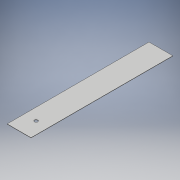
# Autodesk Inventor part: case
Saved by Autodesk Inventor 2019 (Build 230136000, 136)
## iProperties
Created: 2020-03-06
Part Number: case
Material: Generic
Document SubType Name: Sheet Metal
Designer: unusualgamer
Density: 1 g/cm^3
Sheet Metal Rule: Default_mm
Appearance: Default
Author: unusualgamer
Autodesk Inventor part; units mm, degrees
ref_plane "YZ Plane" through (0, 0, 0) normal (1, 0, 0) x (0, 1, 0)
ref_plane "XZ Plane" through (0, 0, 0) normal (0, 1, 0) x (-1, 0, 0)
ref_plane "XY Plane" through (0, 0, 0) normal (0, 0, 1) x (1, 0, 0)
sketch "Sketch1" plane through (0, 0, 0) normal (0, 1, 0) x (-1, 0, 0)
  line L0 (102.7304, -71.3481) -> (60.7304, -71.3481)
  line L1 (60.7304, -71.3481) -> (60.7304, 178.6519)
  line L2 (60.7304, 178.6519) -> (102.7304, 178.6519)
  line L3 (102.7304, 178.6519) -> (102.7304, -71.3481)
  point P0 (0, 0)
  dimension "d0" = 42
  dimension "d1" = 250
  measures "d0" distance of L1.end L2.end
  measures "d1" distance of L0.end L1.end
extrude "Plate1" add sketch "Sketch1" along normal blind 0.5
sketch "Sketch2" plane through (0, 0.5, 0) normal (0, 1, 0) x (1, 0, 0)
  line L0 (-102.7304, -178.6519) -> (-102.7304, 71.3481) projected
  line L1 (-60.7304, -178.6519) -> (-102.7304, -178.6519) projected
  point P0 (0, 0)
  point P1 (-81.7304, -148.6519)
  dimension "d3" = 21
  dimension "d4" = 30
  measures "d3" distance from line of L0 point (-81.73, -148.652)
  measures "d4" distance from line of L1 point (-81.73, -148.652)
hole "Hole1" at (-81.7304, 0.5, 148.6519) direction (0, -1, 0) diameter 6 depth 0.5 tip angle 118
equation "\"d10\" = Thickness"
equation "\"d2\" = Thickness"
equation "\"BendRadius\" = Thickness"
equation "\"BendReliefWidth\" = Thickness"
equation "\"BendReliefDepth\" = 0.5 * Thickness"
equation "\"CornerReliefSize\" = 4 * Thickness"
equation "\"MinimumRemnant\" = 2 * Thickness"
equation "\"TransitionRadius\" = BendRadius"
equation "\"JacobiRadiusSize\" = BendRadius"
equation "\"GapSize\" = Thickness"
equation "\"Thickness\" = 0.5"
body "Solid1"
